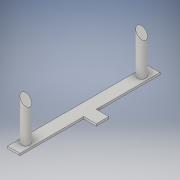
# Autodesk Inventor part: New pi bracket
Saved by Autodesk Inventor 2018 (Build 220112000, 112)
## iProperties
Created: 2019-11-18
Part Number: New pi bracket
Material: Generic
Document SubType Name: Modeling
Designer: Jacob
Density: 1 g/cm^3
Appearance: Default
Author: Jacob
Autodesk Inventor part; units mm, degrees
ref_plane "YZ Plane" through (0, 0, 0) normal (1, 0, 0) x (0, 1, 0)
ref_plane "XZ Plane" through (0, 0, 0) normal (0, 1, 0) x (-1, 0, 0)
ref_plane "XY Plane" through (0, 0, 0) normal (0, 0, 1) x (1, 0, 0)
sketch "Sketch1" plane through (0, 0, 0) normal (0, 1, 0) x (-1, 0, 0)
  line L0 (6, -3) -> (-6, -3)
  line L1 (-6, -3) -> (-6, 3)
  line L2 (-6, 3) -> (6, 3)
  line L3 (6, 3) -> (6, -3)
  line L4 (6, -3) -> (-6, 3) construction
  line L5 (-6, -3) -> (6, 3) construction
  line L6 (3, -3) -> (3, 3) construction
  line L7 (6, -33.5) -> (0, -33.5)
  line L8 (0, -33.5) -> (0, 33.5)
  line L9 (0, 33.5) -> (6, 33.5)
  line L10 (6, 33.5) -> (6, -33.5)
  line L11 (6, -33.5) -> (0, 33.5) construction
  line L12 (0, -33.5) -> (6, 33.5) construction
  line L13 (3, -33.5) -> (3, 33.5) construction
  circle A0 centre (3, 27.7) radius 2
  circle A1 centre (3, -27.7) radius 2
  point P0 (0, 0)
  point P1 (3, 0)
  dimension "d0" = 6
  dimension "d1" = 12
  dimension "d2" = 3
  dimension "d3" = 6
  dimension "d4" = 67
  dimension "d5" = 55.4
  dimension "d6" = 27.7
  dimension "d7" = 27.7
  dimension "d8" = 4
  dimension "d9" = 4
  constraints: 28 end point, 7 midpoint, 4 parallel, 4 point on line, 3 perpendicular, 2 centre point, 2 horizontal
  measures "d0" distance between parallel lines of L2 L0
  measures "d1" distance of L1.end L2.end
  measures "d2" distance between parallel lines of L3 L6
  measures "d3" distance of L7.start L7.end
  measures "d4" distance of L9.end L7.start
  measures "d5" distance of A0.centre A1.centre
  measures "d6" distance of point (3, 0) A1.centre
  measures "d7" distance of point (3, 0) A0.centre
  measures "d8" diameter of A1
  measures "d9" diameter of A0
extrude "Extrusion1" add sketch "Sketch1" along normal blind 1 contours L10 L7 L8 L0 | L0 L8 L2 L3 | L0 L1 L2 L8 | L2 L8 L9 L10 | A0 | A1
sketch "Sketch2" plane through (0, 1, 0) normal (0, 1, 0) x (1, 0, 0)
  line L0 (-6, -33.5) -> (0, -33.5) projected
  line L1 (-3, -33.5) -> (-3, 33.5) construction
  line L2 (-6, 33.5) -> (0, 33.5) projected
  circle A0 centre (-3, -27.7) radius 2
  circle A1 centre (-3, 27.7) radius 2
  line L3 (-6, 0) -> (0, 0) construction
  dimension "d12" = 55.4
  dimension "d13" = 27.7
  dimension "d14" = 27.7
  dimension "d15" = 4
  dimension "d16" = 4
  constraints: 4 end point, 2 centre point, 2 midpoint, 2 point on line, 1 horizontal
  measures "d12" distance of A1.centre A0.centre
  measures "d13" distance from line of L3 A0.centre
  measures "d14" distance from line of L3 A1.centre
  measures "d15" diameter of A0
  measures "d16" diameter of A1
extrude "Extrusion2" add sketch "Sketch2" along normal blind 20
sketch "Sketch3" plane through (-6, 0, 33.5) normal (0, 0, 1) x (1, 0, 0)
  line L0 (5, 21) -> (1, 21) projected
  line L1 (1, 21) -> (8, 21)
  line L2 (8, 21) -> (8, 13.544)
  line L3 (8, 13.544) -> (1, 21)
  point P0 (6, 0)
  dimension "d19" = 7
  constraints: 6 end point, 1 horizontal, 1 perpendicular
  measures "d19" distance of L0.end L1.end
extrude "Extrusion3" cut sketch "Sketch3" against normal blind 100
equation "\"d6\" = d7"
equation "\"d13\" = d14"
body "Solid1"
